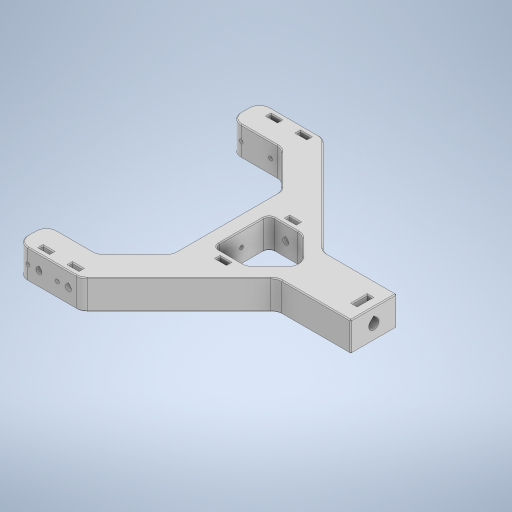
# Autodesk Inventor part: bottom
Saved by Autodesk Inventor 2023.1 (Build 271208000, 208)
## iProperties
Created: 2023-11-14
Part Number: bottom
Material: Generic
Document SubType Name: Modeling
Designer: zavrel
Density: 1 g/cm^3
Appearance: Default
Author: zavrel
Autodesk Inventor part; units mm, degrees
ref_plane "YZ Plane" through (0, 0, 0) normal (1, 0, 0) x (0, 1, 0)
ref_plane "XZ Plane" through (0, 0, 0) normal (0, 1, 0) x (-1, 0, 0)
ref_plane "XY Plane" through (0, 0, 0) normal (0, 0, 1) x (1, 0, 0)
sketch "Sketch1" plane through (0, 0, 0) normal (0, 1, 0) x (-1, 0, 0)
  line L0 (0, 0) -> (0, 12.5)
  line L1 (0, 12.5) -> (40, 12.5)
  line L2 (40, 12.5) -> (93.5, 66)
  line L3 (72, 0) -> (72, 15)
  line L4 (72, 15) -> (53.8137, 15)
  line L5 (53.8137, 15) -> (38.8137, 0)
  line L6 (95.3823, 56.5685) -> (38.8137, 0) construction
  line L7 (80, 29.8726) -> (100.1274, 50)
  line L8 (100.1274, 50) -> (128.1464, 50)
  line L9 (128.1464, 50) -> (128.1464, 66)
  line L10 (128.1464, 66) -> (93.5, 66)
  line L11 (80, 29.8726) -> (80, 0)
  line L12 (0, 0) -> (142.506, 0) construction
  line L13 (0, 0) -> (0, -12.5)
  line L14 (0, -12.5) -> (40, -12.5)
  line L15 (40, -12.5) -> (93.5, -66)
  line L16 (72, 0) -> (72, -15)
  line L17 (72, -15) -> (53.8137, -15)
  line L18 (53.8137, -15) -> (38.8137, 0)
  line L19 (95.3823, -56.5685) -> (38.8137, 0) construction
  line L20 (80, -29.8726) -> (100.1274, -50)
  line L21 (100.1274, -50) -> (128.1464, -50)
  line L22 (128.1464, -50) -> (128.1464, -66)
  line L23 (128.1464, -66) -> (93.5, -66)
  line L24 (80, -29.8726) -> (80, 0)
  point P0 (128.1464, -58)
  point P1 (128.1464, 58)
  dimension "d2" = 40
  dimension "d7" = 45
  dimension "d9" = 8
  dimension "d12" = 16
  dimension "d14" = 30
  dimension "d15" = 25
  dimension "d16" = 8
  dimension "d17" = 116
  dimension "d20" = 16
  constraints: 50 end point, 10 symmetric about line, 4 perpendicular, 3 vertical, 2 horizontal, 2 midpoint, 1 parallel
  measures "d2" distance of L0.end L1.end
  measures "d7" angle of L2 L0
  measures "d9" distance between parallel lines of L5 L2
  measures "d12" distance of L8.end L9.end
  measures "d14" distance between parallel lines of L4 L17
  measures "d15" distance between parallel lines of L14 L1
  measures "d16" distance between parallel lines of L11 L3
  measures "d17" distance of point (128.146, -58) point (128.146, 58)
  measures "d20" distance between parallel lines of L2 L7
extrude "Extrusion1" add sketch "Sketch1" along normal blind 16
sketch "Sketch2" plane through (-80, 0, -29.8726) normal (-1, 0, 0) x (0, 0, 1)
  line L0 (0, 0) -> (59.7452, 0) projected
  line L1 (59.7452, 0) -> (59.7452, 16) projected
  line L2 (0, 16) -> (59.7452, 16) projected
  line L3 (0, 0) -> (0, 16) projected
  line L4 (0, 0) -> (59.7452, 0) construction
  line L5 (59.7452, 0) -> (0, 16) construction
  line L6 (0, 0) -> (0, 16) construction
  line L7 (0, 0) -> (59.7452, 16) construction
  circle A0 centre (29.8726, 8) radius 1
  point P0 (29.8726, 0)
  dimension "d21" = 2
  constraints: 4 end point, 1 centre point, 1 midpoint
  measures "d21" diameter of A0
extrude "Extrusion2" cut sketch "Sketch2" against normal up to surface (8 mm away) contours A0
sketch "Sketch3" plane through (0, 16, 0) normal (0, 1, 0) x (1, 0, 0)
  line L0 (-40, 12.5) -> (-93.5, 66) projected
  line L1 (-93.5, 66) -> (-128.1464, 66) projected
  line L2 (-128.1464, 66) -> (-128.1464, 50) projected
  line L3 (-128.1464, 50) -> (-100.1274, 50) projected
  line L4 (-100.1274, 50) -> (-80, 29.8726) projected
  line L5 (-80, 29.8726) -> (-80, -29.8726) projected
  line L6 (-80, -29.8726) -> (-100.1274, -50) projected
  line L7 (-100.1274, -50) -> (-128.1464, -50) projected
  line L8 (-128.1464, -50) -> (-128.1464, -66) projected
  line L9 (-128.1464, -66) -> (-93.5, -66) projected
  line L10 (-93.5, -66) -> (-40, -12.5) projected
  line L11 (-40, -12.5) -> (0, -12.5) projected
  line L12 (0, -12.5) -> (0, 12.5) projected
  line L13 (0, 12.5) -> (-40, 12.5) projected
  line L14 (-72, 15) -> (-53.8137, 15) projected
  line L15 (-53.8137, 15) -> (-38.8137, 0) projected
  line L16 (-38.8137, 0) -> (-53.8137, -15) projected
  line L17 (-53.8137, -15) -> (-72, -15) projected
  line L18 (-72, -15) -> (-72, 15) projected
  line L19 (-53.8137, -15) -> (-72, -15) construction
  line L20 (-62.9069, -15) -> (-62.9069, 15) construction
  line L21 (-72, 15) -> (-53.8137, 15) construction
  line L22 (-65.6569, -20) -> (-60.1569, -20)
  line L23 (-60.1569, -20) -> (-60.1569, -18)
  line L24 (-60.1569, -18) -> (-65.6569, -18)
  line L25 (-65.6569, -18) -> (-65.6569, -20)
  line L26 (-72, -15) -> (-72, 15) construction
  line L27 (-72, 0) -> (-38.8137, 0) construction
  line L28 (-65.6569, 20) -> (-60.1569, 20)
  line L29 (-60.1569, 20) -> (-60.1569, 18)
  line L30 (-60.1569, 18) -> (-65.6569, 18)
  line L31 (-65.6569, 18) -> (-65.6569, 20)
  point P0 (0, 0)
  point P1 (-62.9069, -18)
  point P2 (-62.9069, 18)
  dimension "d24" = 5.5
  dimension "d25" = 2
  dimension "d26" = 3
  constraints: 20 end point, 5 symmetric about line, 4 midpoint, 2 parallel, 2 perpendicular, 1 horizontal, 1 point on line
  measures "d24" distance of L23.end L24.end
  measures "d25" distance of L22.end L23.end
  measures "d26" distance between parallel lines of L17 L24
extrude "Extrusion3" cut sketch "Sketch3" against normal blind 11 contours L25 L24 L23 L22 | L28 L29 L30 L31
sketch "Sketch4" plane through (-53.8137, 0, 15) normal (0, 0, -1) x (-1, 0, 0)
  line L0 (0, 0) -> (18.1863, 0) projected
  line L1 (18.1863, 0) -> (18.1863, 16) projected
  line L2 (0, 16) -> (18.1863, 16) projected
  line L3 (0, 0) -> (0, 16) projected
  line L4 (18.1863, 16) -> (0, 0) construction
  line L5 (18.1863, 0) -> (0, 16) construction
  circle A0 centre (9.0931, 8) radius 1.6
  line L6 (9.0931, 8) -> (9.0931, 14.2049) construction
  line L7 (9.0931, 10.2627) -> (10.2245, 9.1314)
  line L8 (9.0931, 10.2627) -> (7.9618, 9.1314)
  point P0 (-53.8137, 0)
  dimension "d29" = 3.2
  dimension "d30" = 90
  constraints: 10 end point, 2 point on circle, 2 tangent, 1 centre point, 1 midpoint, 1 point on line, 1 vertical
  measures "d29" diameter of A0
  measures "d30" angle of L8 L7
extrude "Extrusion4" cut sketch "Sketch4" against normal blind 12 contours A0 | A0 L8 L7
sketch "Sketch5" plane through (-72, 0, -15) normal (0, 0, 1) x (1, 0, 0)
  line L0 (0, 0) -> (18.1863, 0) projected
  line L1 (18.1863, 0) -> (18.1863, 16) projected
  line L2 (0, 16) -> (18.1863, 16) projected
  line L3 (0, 0) -> (0, 16) projected
  line L4 (0, 0) -> (18.1863, 0)
  line L5 (18.1863, 0) -> (18.1863, 16)
  line L6 (0, 16) -> (18.1863, 16)
  line L7 (0, 0) -> (0, 16)
  line L8 (18.1863, 16) -> (0, 0) construction
  line L9 (18.1863, 0) -> (0, 16) construction
  circle A0 centre (9.0931, 8) radius 1.6
  line L10 (9.0931, 8) -> (9.0931, 14.2049) construction
  line L11 (9.0931, 10.2627) -> (10.2245, 9.1314)
  line L12 (9.0931, 10.2627) -> (7.9618, 9.1314)
  point P0 (72, 0)
  point P1 (-53.8137, 0)
  dimension "d33" = 3.2
  dimension "d34" = 90
  constraints: 18 end point, 2 point on circle, 2 tangent, 1 centre point, 1 midpoint, 1 point on line, 1 vertical
  measures "d33" diameter of A0
  measures "d34" angle of L12 L11
extrude "Extrusion5" cut sketch "Sketch5" against normal blind 12 contours A0 | A0 L12 L11
sketch "Sketch7" plane through (0, 0, 12.5) normal (1, 0, 0) x (0, 0, -1)
  line L0 (0, 0) -> (25, 0) projected
  line L1 (25, 0) -> (25, 16) projected
  line L2 (0, 16) -> (25, 16) projected
  line L3 (0, 0) -> (0, 16) projected
  line L4 (0, 16) -> (25, 16) construction
  line L5 (0, 16) -> (25, 0) construction
  line L6 (25, 16) -> (0, 0) construction
  line L7 (12.5, 0) -> (12.5, 16) projected
  circle A0 centre (12.5, 8) radius 2.75
  line L8 (12.5, 11.8891) -> (10.5555, 9.9445)
  line L9 (12.5, 11.8891) -> (14.4445, 9.9445)
  dimension "d37" = 5.5
  dimension "d45" = 90
  constraints: 8 end point, 2 point on circle, 2 tangent, 1 centre point, 1 midpoint, 1 point on line
  measures "d37" diameter of A0
  measures "d45" angle of L9 L8
extrude "Extrusion6" cut sketch "Sketch7" against normal blind 20 contours A0 L7 | L7 A0 | A0 L8 L7 | L7 L9 A0
sketch "Sketch8" plane through (0, 16, 0) normal (0, 1, 0) x (1, 0, 0)
  line L0 (-60.1569, 18) -> (-65.6569, 18) projected
  line L1 (-65.6569, 18) -> (-65.6569, 20) projected
  line L2 (-65.6569, 20) -> (-60.1569, 20) projected
  line L3 (-60.1569, 20) -> (-60.1569, 18) projected
  line L4 (-65.6569, -18) -> (-60.1569, -18) projected
  line L5 (-60.1569, -18) -> (-60.1569, -20) projected
  line L6 (-60.1569, -20) -> (-65.6569, -20) projected
  line L7 (-65.6569, -20) -> (-65.6569, -18) projected
  line L8 (-40, 12.5) -> (-93.5, 66) projected
  line L9 (-93.5, 66) -> (-128.1464, 66) projected
  line L10 (-128.1464, 66) -> (-128.1464, 50) projected
  line L11 (-128.1464, 50) -> (-100.1274, 50) projected
  line L12 (-100.1274, 50) -> (-80, 29.8726) projected
  line L13 (-80, 29.8726) -> (-80, -29.8726) projected
  line L14 (-80, -29.8726) -> (-100.1274, -50) projected
  line L15 (-100.1274, -50) -> (-128.1464, -50) projected
  line L16 (-128.1464, -50) -> (-128.1464, -66) projected
  line L17 (-128.1464, -66) -> (-93.5, -66) projected
  line L18 (-93.5, -66) -> (-40, -12.5) projected
  line L19 (-40, -12.5) -> (0, -12.5) projected
  line L20 (0, -12.5) -> (0, 12.5) projected
  line L21 (0, 12.5) -> (-40, 12.5) projected
  line L22 (-72, 15) -> (-53.8137, 15) projected
  line L23 (-53.8137, 15) -> (-38.8137, 0) projected
  line L24 (-38.8137, 0) -> (-53.8137, -15) projected
  line L25 (-53.8137, -15) -> (-72, -15) projected
  line L26 (-72, -15) -> (-72, 15) projected
  line L27 (-7.6, -4) -> (-5, -4)
  line L28 (-5, -4) -> (-5, 4)
  line L29 (-5, 4) -> (-7.6, 4)
  line L30 (-7.6, 4) -> (-7.6, -4)
  line L31 (-53.8137, 15) -> (-38.8137, 0) construction
  line L32 (0, 0) -> (-38.8137, 0) construction
  point P0 (-5, 0)
  dimension "d40" = 2.6
  dimension "d41" = 5
  dimension "d42" = 8
  constraints: 10 end point, 2 horizontal, 2 parallel, 1 midpoint, 1 perpendicular, 1 point on line
  measures "d40" distance between parallel lines of L28 L30
  measures "d41" distance between parallel lines of L20 L28
  measures "d42" distance between parallel lines of L27 L29
extrude "Extrusion7" cut sketch "Sketch8" against normal blind 13 contours L30 L29 L28 L27
sketch "Sketch9" plane through (-100.1274, 0, 50) normal (0, 0, -1) x (-1, 0, 0)
  line L0 (0, 0) -> (28.019, 0) projected
  line L1 (28.019, 0) -> (28.019, 16) projected
  line L2 (0, 16) -> (28.019, 16) projected
  line L3 (0, 0) -> (0, 16) projected
  line L4 (28.019, 0) -> (28.019, 16) construction
  line L5 (28.019, 8) -> (0, 8) construction
  circle A0 centre (22.019, 8) radius 1
  circle A1 centre (6.019, 8) radius 1
  point P0 (-100.1274, 0)
  dimension "d46" = 2
  dimension "d47" = 2
  dimension "d48" = 6
  dimension "d49" = 16
  constraints: 2 centre point, 2 end point, 2 midpoint, 2 point on line
  measures "d46" diameter of A1
  measures "d47" diameter of A0
  measures "d48" distance from line of L1 A0.centre
  measures "d49" distance of A0.centre A1.centre
extrude "Extrusion8" cut sketch "Sketch9" against normal through all contours A0 | A1
sketch "Sketch11" plane through (-128.1464, 0, 66) normal (0, 0, 1) x (1, 0, 0)
  circle A0 centre (22, 8) radius 1 projected
  circle A1 centre (6, 8) radius 1 projected
  line L0 (0, 0) -> (34.6464, 0) projected
  line L1 (34.6464, 0) -> (34.6464, 16) projected
  line L2 (0, 16) -> (34.6464, 16) projected
  line L3 (0, 0) -> (0, 16) projected
  circle A2 centre (12, 8) radius 1.5999
  line L4 (12, 8) -> (12, 11.5478) construction
  line L5 (12, 10.2626) -> (10.8687, 9.1313)
  line L6 (12, 10.2626) -> (13.1313, 9.1313)
  circle A3 centre (28, 8) radius 1.5999
  line L7 (28, 8) -> (28, 11.5478) construction
  line L8 (28, 10.2626) -> (26.8687, 9.1313)
  line L9 (28, 10.2626) -> (29.1313, 9.1313)
  point P0 (128.1464, 0)
  dimension "d52" = 6
  dimension "d54" = 90
  dimension "d55" = 90
  dimension "d56" = 6
  constraints: 12 end point, 4 point on circle, 4 tangent, 2 centre point, 2 point on line, 2 vertical
  measures "d52" distance of L4.start A1.centre
  measures "d54" angle of L6 L5
  measures "d55" angle of L9 L8
  measures "d56" distance of A0.centre L7.start
extrude "Extrusion9" cut sketch "Sketch11" against normal blind 12 contours A2 | A2 L5 L6 | A3 | A3 L8 L9
sketch "Sketch12" plane through (-128.1464, 0, -50) normal (0, 0, 1) x (1, 0, 0)
  line L0 (0, 0) -> (28.019, 0)
  line L1 (28.019, 0) -> (28.019, 16)
  line L2 (0, 16) -> (28.019, 16)
  line L3 (0, 0) -> (0, 16)
  line L4 (28.019, 0) -> (28.019, 16) construction
  line L5 (28.019, 8) -> (0, 8) construction
  circle A0 centre (22.019, 8) radius 1
  circle A1 centre (6.019, 8) radius 1
  point P0 (128.1464, 0)
  point P1 (-100.1274, 0)
  dimension "d59" = 2
  dimension "d60" = 2
  dimension "d61" = 6
  dimension "d62" = 16
  constraints: 12 end point, 2 centre point, 2 midpoint, 2 point on line
  measures "d59" diameter of A1
  measures "d60" diameter of A0
  measures "d61" distance from line of L1 A0.centre
  measures "d62" distance of A0.centre A1.centre
extrude "Extrusion10" cut sketch "Sketch12" against normal through all contours A0 | A1
sketch "Sketch14" plane through (-93.5, 0, -66) normal (0, 0, -1) x (-1, 0, 0)
  circle A0 centre (6.6274, 8) radius 1.5999
  line L0 (6.6274, 8) -> (6.6274, 9.8664) construction
  line L1 (6.6274, 10.2626) -> (5.4961, 9.1313)
  line L2 (6.6274, 10.2626) -> (7.7587, 9.1313)
  circle A1 centre (22.6274, 8) radius 1.5999
  line L3 (22.6274, 8) -> (22.6274, 10.5588) construction
  line L4 (22.6274, 10.2626) -> (21.4961, 9.1313)
  line L5 (22.6274, 10.2626) -> (23.7587, 9.1313)
  circle A2 centre (12.6274, 8) radius 1 projected
  circle A3 centre (28.6274, 8) radius 1 projected
  line L6 (0, 0) -> (34.6464, 0) projected
  line L7 (34.6464, 0) -> (34.6464, 16) projected
  line L8 (0, 16) -> (34.6464, 16) projected
  line L9 (0, 0) -> (0, 16) projected
  line L10 (34.6464, 0) -> (34.6464, 16) construction
  line L11 (34.6464, 8) -> (0, 8) construction
  point P0 (-93.5, 0)
  point P1 (128.1464, 0)
  dimension "d70" = 90
  dimension "d71" = 90
  dimension "d73" = 3.1999
  dimension "d74" = 6
  dimension "d75" = 6
  constraints: 14 end point, 4 point on circle, 4 point on line, 4 tangent, 2 centre point, 2 midpoint, 2 vertical
  measures "d70" angle of L2 L1
  measures "d71" angle of L5 L4
  measures "d73" diameter of A1
  measures "d74" distance of A3.centre L3.start
  measures "d75" distance of A2.centre L0.start
extrude "Extrusion11" cut sketch "Sketch14" against normal blind 12 contours A0 | A0 L1 L2 | A1 | A1 L4 L5
sketch "Sketch15" plane through (0, 16, 0) normal (0, 1, 0) x (1, 0, 0)
  line L0 (-7.6, 4) -> (-5, 4) projected
  line L1 (-5, 4) -> (-5, -4) projected
  line L2 (-5, -4) -> (-7.6, -4) projected
  line L3 (-7.6, -4) -> (-7.6, 4) projected
  line L4 (-60.1569, 18) -> (-65.6569, 18) projected
  line L5 (-65.6569, 18) -> (-65.6569, 20) projected
  line L6 (-65.6569, 20) -> (-60.1569, 20) projected
  line L7 (-60.1569, 20) -> (-60.1569, 18) projected
  line L8 (-65.6569, -18) -> (-60.1569, -18) projected
  line L9 (-60.1569, -18) -> (-60.1569, -20) projected
  line L10 (-60.1569, -20) -> (-65.6569, -20) projected
  line L11 (-65.6569, -20) -> (-65.6569, -18) projected
  line L12 (-40, 12.5) -> (-93.5, 66) projected
  line L13 (-93.5, 66) -> (-128.1464, 66) projected
  line L14 (-128.1464, 66) -> (-128.1464, 50) projected
  line L15 (-128.1464, 50) -> (-100.1274, 50) projected
  line L16 (-100.1274, 50) -> (-80, 29.8726) projected
  line L17 (-80, 29.8726) -> (-80, -29.8726) projected
  line L18 (-80, -29.8726) -> (-100.1274, -50) projected
  line L19 (-100.1274, -50) -> (-128.1464, -50) projected
  line L20 (-128.1464, -50) -> (-128.1464, -66) projected
  line L21 (-128.1464, -66) -> (-93.5, -66) projected
  line L22 (-93.5, -66) -> (-40, -12.5) projected
  line L23 (-40, -12.5) -> (0, -12.5) projected
  line L24 (0, -12.5) -> (0, 12.5) projected
  line L25 (0, 12.5) -> (-40, 12.5) projected
  line L26 (-72, 15) -> (-53.8137, 15) projected
  line L27 (-53.8137, 15) -> (-38.8137, 0) projected
  line L28 (-38.8137, 0) -> (-53.8137, -15) projected
  line L29 (-53.8137, -15) -> (-72, -15) projected
  line L30 (-72, -15) -> (-72, 15) projected
  line L31 (-80, 29.8726) -> (-80, -29.8726) construction
  line L32 (-80, 0) -> (-72, 0) construction
  line L33 (-118.8964, -63) -> (-113.3964, -63)
  line L34 (-113.3964, -63) -> (-113.3964, -61)
  line L35 (-113.3964, -61) -> (-118.8964, -61)
  line L36 (-118.8964, -61) -> (-118.8964, -63)
  line L37 (-102.8964, -63) -> (-97.3964, -63)
  line L38 (-97.3964, -63) -> (-97.3964, -61)
  line L39 (-97.3964, -61) -> (-102.8964, -61)
  line L40 (-102.8964, -61) -> (-102.8964, -63)
  line L41 (-118.8964, 63) -> (-113.3964, 63)
  line L42 (-113.3964, 63) -> (-113.3964, 61)
  line L43 (-113.3964, 61) -> (-118.8964, 61)
  line L44 (-118.8964, 61) -> (-118.8964, 63)
  line L45 (-102.8964, 63) -> (-97.3964, 63)
  line L46 (-97.3964, 63) -> (-97.3964, 61)
  line L47 (-97.3964, 61) -> (-102.8964, 61)
  line L48 (-102.8964, 61) -> (-102.8964, 63)
  point P0 (0, 0)
  point P1 (-116.1464, -63)
  point P2 (-100.1464, -63)
  point P3 (-116.1464, 63)
  point P4 (-100.1464, 63)
  dimension "d78" = 2
  dimension "d79" = 5.5
  dimension "d80" = 3
  dimension "d81" = 12
  dimension "d82" = 16
  constraints: 34 end point, 10 symmetric about line, 4 midpoint, 4 parallel, 2 equal length, 2 horizontal, 2 perpendicular, 2 point on line
  measures "d78" distance of L35.end L33.start
  measures "d79" distance of L34.end L35.end
  measures "d80" distance between parallel lines of L21 L33
  measures "d81" distance from line of L20 point (-116.146, -63)
  measures "d82" distance of point (-100.146, -63) point (-116.146, -63)
extrude "Extrusion12" cut sketch "Sketch15" against normal blind 11 contours L36 L35 L34 L33 | L40 L39 L38 L37 | L41 L42 L43 L44 | L45 L46 L47 L48
fillet "Fillet1" radius 6 15 edges at (-53.8137, 8, 15) (-38.8137, 8, 0) (-53.8137, 8, -15) (-40, 8, -12.5) (-40, 8, 12.5) (-93.5, 8, 66) (-100.1274, 8, -50) (-100.1274, 8, 50) (-80, 8, 29.8726) (-80, 8, -29.8726) (-93.5, 8, -66) (-128.1464, 8, -66) (-128.1464, 8, -50) (-128.1464, 8, 66) (-128.1464, 8, 50)
fillet "Fillet2" radius 3 2 edges at (-72, 8, 15) (-72, 8, -15)
chamfer "Chamfer1" distance 0.5 angle 45 84 edges at (-66.75, 16, 39.25) (-93.6892, 16, 65.5433) (-18.7574, 16, 12.5) (-109.0659, 16, 66) (-126.3891, 16, 64.2426) (-128.1464, 16, 58) (-126.3891, 16, 51.7574) (-112.3796, 16, 50) (-90.0637, 16, 39.9363) (-126.3891, 16, -51.7574) (-126.3891, 16, -64.2426) (-93.6892, 16, -65.5433) (-80, 16, 0) (-90.0637, 16, -39.9363) (-112.3796, 16, -50) (-128.1464, 16, -58) (-109.0659, 16, -66) (-66.75, 16, -39.25) (-18.7574, 16, -12.5) (-66.75, 0, 39.25) (-93.6892, 0, 65.5433) (-18.7574, 0, 12.5) (-109.0659, 0, 66) (-126.3891, 0, 64.2426) (-128.1464, 0, 58) (-126.3891, 0, 51.7574) (-112.3796, 0, 50) (-90.0637, 0, 39.9363) (-126.3891, 0, -51.7574) (-126.3891, 0, -64.2426) (-93.6892, 0, -65.5433) (-80, 0, 0) (-90.0637, 0, -39.9363) (-112.3796, 0, -50) (-128.1464, 0, -58) (-109.0659, 0, -66) (-66.75, 0, -39.25) (-18.7574, 0, -12.5) (-62.6495, 16, 15) (-71.1213, 16, 14.1213) (-72, 16, 0) (-71.1213, 16, -14.1213) (-62.6495, 16, -15) (-47.5563, 16, -8.7426) (-47.5563, 16, 8.7426) (-72, 0, 0) (-71.1213, 0, -14.1213) (-62.6495, 0, -15) (-47.5563, 0, -8.7426) (-47.5563, 0, 8.7426) (-62.6495, 0, 15) (-71.1213, 0, 14.1213) (-116.1464, 16, 61) (-118.8964, 16, 62) (-116.1464, 16, 63) (-113.3964, 16, 62) (-102.8964, 16, 62) (-100.1464, 16, 63) (-100.1464, 16, 61) (-97.3964, 16, 62) (-62.9069, 16, 20) (-65.6569, 16, 19) (-62.9069, 16, 18) (-60.1569, 16, 19) (-62.9069, 16, -20) (-62.9069, 16, -18) (-65.6569, 16, -19) (-60.1569, 16, -19) (-7.6, 16, 0) (-6.3, 16, 4) (-5, 16, 0) (-6.3, 16, -4) (-116.1464, 16, -63) (-118.8964, 16, -62) (-116.1464, 16, -61) (-113.3964, 16, -62) (-102.8964, 16, -62) (-100.1464, 16, -61) (-100.1464, 16, -63) (-97.3964, 16, -62) (0, 16, 0) (0, 8, 12.5) (0, 0, 0) (0, 8, -12.5)
body "Solid1"
